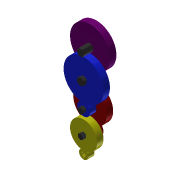
# Autodesk Inventor part: Gearbox Mockup
Saved by Autodesk Inventor 2015 (Build 190159000, 159)
## iProperties
Created: 2014-11-29
Part Number: Gearbox Mockup
Material: Generic
Document SubType Name: Modeling
Designer: Nemo
Density: 1 g/cm^3
Appearance: Default
Author: Nemo
Autodesk Inventor part; units mm, degrees
note: some values were not read from the file. Chosen so that the rebuilt part matches the saved one: sketch regions of "Extrusion2"; sketch regions of "Extrusion4"; sketch regions of "Extrusion5"; sketch regions of "Extrusion6".
ref_plane "YZ Plane" through (0, 0, 0) normal (1, 0, 0) x (0, 1, 0)
ref_plane "XZ Plane" through (0, 0, 0) normal (0, 1, 0) x (-1, 0, 0)
ref_plane "XY Plane" through (0, 0, 0) normal (0, 0, 1) x (1, 0, 0)
sketch "Sketch1" plane through (0, 0, 0) normal (0, 0, 1) x (1, 0, 0)
  circle A0 centre (0, 0) radius 7.62
  circle A1 centre (0, 0) radius 31.75 construction
  circle A2 centre (0, 0) radius 8.89
  circle A3 centre (0, 33.0962) radius 25.4
  circle A4 centre (0, 33.0962) radius 12.7
  circle A5 centre (0, 77.6224) radius 31.75
  circle A6 centre (0, 77.6224) radius 11.43
  circle A7 centre (0, 127.2286) radius 38.1
  circle A8 centre (0, 127.2286) radius 11.43
  circle A9 centre (0, 176.8348) radius 38.1
  circle A10 centre (0, 33.0962) radius 13.97
  circle A11 centre (0, 33.0962) radius 26.67
  circle A12 centre (0, 77.6224) radius 12.7
  circle A13 centre (0, 77.6224) radius 33.02
  circle A14 centre (0, 127.2286) radius 12.7
  circle A15 centre (0, 127.2286) radius 39.37
  circle A16 centre (0, 176.8348) radius 39.37
  line L0 (0, 38.5955) -> (4.7625, 35.8458)
  line L1 (4.7625, 35.8458) -> (4.7625, 30.3466)
  line L2 (4.7625, 30.3466) -> (0, 27.5969)
  line L3 (0, 27.5969) -> (-4.7625, 30.3466)
  line L4 (-4.7625, 30.3466) -> (-4.7625, 35.8458)
  line L5 (-4.7625, 35.8458) -> (0, 38.5955)
  line L6 (0, 83.1217) -> (4.7625, 80.372)
  line L7 (4.7625, 80.372) -> (4.7625, 74.8728)
  line L8 (4.7625, 74.8728) -> (0, 72.1231)
  line L9 (0, 72.1231) -> (-4.7625, 74.8728)
  line L10 (-4.7625, 74.8728) -> (-4.7625, 80.372)
  line L11 (-4.7625, 80.372) -> (0, 83.1217)
  line L12 (0, 134.5609) -> (6.35, 130.8948)
  line L13 (6.35, 130.8948) -> (6.35, 123.5624)
  line L14 (6.35, 123.5624) -> (0, 119.8963)
  line L15 (0, 119.8963) -> (-6.35, 123.5624)
  line L16 (-6.35, 123.5624) -> (-6.35, 130.8948)
  line L17 (-6.35, 130.8948) -> (0, 134.5609)
  line L18 (3.6662, 183.1848) -> (7.3323, 176.8348)
  line L19 (7.3323, 176.8348) -> (3.6662, 170.4848)
  line L20 (3.6662, 170.4848) -> (-3.6662, 170.4848)
  line L21 (-3.6662, 170.4848) -> (-7.3323, 176.8348)
  line L22 (-7.3323, 176.8348) -> (-3.6662, 183.1848)
  line L23 (-3.6662, 183.1848) -> (3.6662, 183.1848)
  circle A17 centre (0, 0) radius 3.9751
  line L24 (-1, -1.9265) -> (1, -1.9265)
  line L25 (1, -1.9265) -> (1, -5.768)
  line L26 (1, -5.768) -> (-1, -5.768)
  line L27 (-1, -5.768) -> (-1, -1.9265)
  point P0 (-1, -3.8473)
  point P1 (1, -3.8473)
  point P2 (0, -5.768)
  dimension "d0" = 15.24
  dimension "d1" = 63.5
  dimension "d2" = 17.78
  dimension "d3" = 50.8
  dimension "d4" = 33.0962
  dimension "d5" = 25.4
  dimension "d6" = 63.5
  dimension "d7" = 44.5262
  dimension "d8" = 22.86
  dimension "d9" = 76.2
  dimension "d10" = 49.6062
  dimension "d11" = 22.86
  dimension "d12" = 76.2
  dimension "d13" = 49.6062
  dimension "d14" = 27.94
  dimension "d15" = 53.34
  dimension "d18" = 25.4
  dimension "d19" = 66.04
  dimension "d20" = 25.4
  dimension "d21" = 78.74
  dimension "d22" = 78.74
  dimension "d23" = 9.525
  dimension "d24" = 12.7
  dimension "d25" = 7.9502
  dimension "d26" = 2
  dimension "d39" = 12.7
  constraints: 56 end point, 19 coincident, 18 centre point, 8 vertical alignment, 3 midpoint, 2 parallel, 2 point on circle, 1 collinear, 1 horizontal, 1 horizontal alignment, 1 perpendicular, 52 other
  measures "d0" diameter of A0
  measures "d1" diameter of A1
  measures "d2" diameter of A2
  measures "d3" diameter of A3
  measures "d4" distance of point (0, 0) A3.centre
  measures "d5" diameter of A4
  measures "d6" diameter of A5
  measures "d7" distance of A3.centre A5.centre
  measures "d8" diameter of A6
  measures "d9" diameter of A7
  measures "d10" distance of A5.centre A7.centre
  measures "d11" diameter of A8
  measures "d12" diameter of A9
  measures "d13" distance of A7.centre A9.centre
  measures "d14" diameter of A10
  measures "d15" diameter of A11
  measures "d18" diameter of A12
  measures "d19" diameter of A13
  measures "d20" diameter of A14
  measures "d21" diameter of A15
  measures "d22" diameter of A16
  measures "d23" distance between parallel lines of L4 L1
  measures "d24" distance between parallel lines of L20 L23
  measures "d25" diameter of A17
  measures "d26" distance of L25.end L26.end
  measures "d39" distance between parallel lines of L13 L16
extrude "Extrusion2" add sketch "Sketch1" along normal blind 12.7 contours A0 A11 | A0 A11 A2 | A11 A0 | A0 A11 A2 A3 | A2 A3 A13 A11 | A11 A13 A3 A2 | A3 A2 | A2 A3 A13 A10 | A11 A5 A3 A13 | A13 A3 A5 A11 | A3 A5 A10 A13 | A11 A5 A3 | A13 A10 A5 A3 | A3 A5 A10 | A13 A4 A10 | A10 A5 A13 A4 | A10 A5 | A13 A4 | A4 A13
extrude "Extrusion4" add sketch "Sketch1" against normal blind 12.7 separate body contours A13 A15 A5 A11 | A11 A5 A3 A13 | A13 A3 A5 A11 | A11 A5 A15 A13 | A3 A5 A10 A13 | A11 A5 A3 | A5 A15 A12 A11 | A13 A7 A5 A15 | A13 A10 A5 A3 | A3 A5 A10 | A13 A4 A10 | A10 A5 A13 A4 | A5 A7 A12 A15 | A13 A7 A5 | A15 A5 A7 A13 | A10 A5 | A13 A4 | A4 A13 | A5 A7 A12 | A15 A6 A12 | A12 A7 A15 A6 | A15 A12 A7 A5 | A12 A7 | A15 A6 | A6 A15
extrude "Extrusion5" add sketch "Sketch1" along normal blind 12.7 separate body contours A15 A16 A7 A13 | A13 A7 A5 A15 | A5 A7 A12 A15 | A13 A7 A5 | A7 A16 A14 A13 | A15 A9 A7 A16 | A15 A5 A7 A13 | A13 A7 A16 A15 | A5 A7 A12 | A15 A6 A12 | A12 A7 A15 A6 | A7 A9 A14 A16 | A15 A9 A7 | A15 A12 A7 A5 | A12 A7 | A15 A6 | A6 A15 | A7 A9 A14 | A16 A8 A14 | A14 A9 A16 A8 | A15 A16 A7 A9 | A7 A16 A14 A9 | A14 A9 | A16 A8 | A8 A16
extrude "Extrusion6" add sketch "Sketch1" against normal blind 12.7 separate body contours A16 A15 A9 | A15 A9 A7 A16 | A7 A9 A14 A16 | A15 A9 A7 | A9 A15 | A7 A9 A14 | A16 A8 A14 | A14 A9 A16 A8 | A15 A16 A7 A9 | A7 A16 A14 A9 | A14 A9 | A16 A8 | A8 A16
extrude "Extrusion7" add sketch "Sketch1" along normal mid plane 38.1 separate body contours L0 L1 L2 L3 L4 L5 | L6 L7 L8 L9 L10 L11 | L12 L13 L14 L15 L16 L17 | L18 L19 L20 L21 L22 L23
equation "\"d0\" = 0.05 * S1in"
equation "\"d3\" = 0.05 * S1out"
equation "\"d5\" = 0.05 * S2in"
equation "\"d6\" = 0.05 * S2out"
equation "\"d8\" = 0.05 * S3in"
equation "\"d9\" = 0.05 * S3out"
equation "\"d11\" = 0.05 * S4in"
equation "\"d12\" = 0.05 * S4out"
equation "\"S1in\" = 304.8"
equation "\"S1out\" = 1016"
equation "\"S2in\" = 508"
equation "\"S3in\" = 457.2"
equation "\"S3out\" = 1524"
equation "\"S4in\" = 457.2"
equation "\"S4out\" = 1524"
equation "\"S2out\" = 1270"
